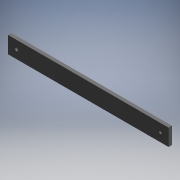
# Autodesk Inventor part: bar arms
Saved by Autodesk Inventor 2019 (Build 230136000, 136)
## iProperties
Part Number: bar arms
Material: Generic
Document SubType Name: Modeling
Designer: Delta
Appearance: Default
Author: Delta
Autodesk Inventor part; units mm, degrees
ref_plane "YZ Plane" through (0, 0, 0) normal (1, 0, 0) x (0, 1, 0)
ref_plane "XZ Plane" through (0, 0, 0) normal (0, 1, 0) x (-1, 0, 0)
ref_plane "XY Plane" through (0, 0, 0) normal (0, 0, 1) x (1, 0, 0)
sketch "Sketch1" plane through (0, 0, 0) normal (0, 0, 1) x (1, 0, 0)
  line L0 (0, 0) -> (304.8, 0)
  line L1 (304.8, 0) -> (304.8, 31.75)
  line L2 (304.8, 31.75) -> (0, 31.75)
  line L3 (0, 31.75) -> (0, 0)
  dimension "d0" = 304.8
  dimension "d1" = 31.75
  constraints: 8 end point, 2 parallel, 1 horizontal, 1 perpendicular
  measures "d0" distance of L2.end L1.end
  measures "d1" distance of L1.end L0.end
extrude "Extrusion1" add sketch "Sketch1" along normal blind 6.35
sketch "Sketch2" plane through (0, 0, 6.35) normal (0, 0, 1) x (1, 0, 0)
  line L0 (0, 31.75) -> (0, 0) projected
  line L1 (0, 0) -> (304.8, 0) projected
  line L2 (304.8, 31.75) -> (0, 31.75) projected
  circle A0 centre (15.875, 15.875) radius 2.8829
  dimension "d4" = 15.875
  dimension "d5" = 31.75
  dimension "d6" = 5.7658
  dimension "d15" = 15.875
  constraints: 1 centre point, 1 coincident
  measures "d4" distance from line of L0 point (15.875, 15.875)
  measures "d5" distance between parallel lines of L1 L2
  measures "d6" diameter of A0
  measures "d15" distance from line of L2 A0.centre
extrude "Extrusion2" cut sketch "Sketch2" against normal through all
sketch "Sketch3" plane through (0, 0, 6.35) normal (0, 0, 1) x (1, 0, 0)
  line L0 (0, 0) -> (304.8, 0) projected
  line L1 (304.8, 31.75) -> (0, 31.75) projected
  line L2 (304.8, 0) -> (304.8, 31.75) projected
  circle A0 centre (288.925, 15.875) radius 2.54
  dimension "d9" = 31.75
  dimension "d10" = 15.875
  dimension "d11" = 15.875
  dimension "d12" = 5.08
  constraints: 1 centre point, 1 coincident
  measures "d9" distance between parallel lines of L0 L1
  measures "d10" distance from line of L2 point (288.925, 15.875)
  measures "d11" distance from line of L1 point (288.925, 15.875)
  measures "d12" diameter of A0
extrude "Extrusion3" cut sketch "Sketch3" against normal through all
equation "\"d4\" = 0.5 * d5"
equation "\"d15\" = 0.5 * d5"
equation "\"d10\" = 0.5 * d9"
equation "\"d11\" = 0.5 * d9"
body "Solid1"
